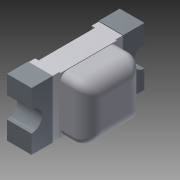
# Autodesk Inventor part: 0603_led
Saved by Autodesk Inventor 2013 (Build 170138000, 138)
## iProperties
Created: 2015-03-28
Part Number: 0603_led
Material: Ogólny
Document SubType Name: Modeling
Designer: terg
Density: 1 g/cm^3
Author: terg
Autodesk Inventor part; units mm, degrees
ref_plane "YZ Plane" through (0, 0, 0) normal (1, 0, 0) x (0, 1, 0)
ref_plane "XZ Plane" through (0, 0, 0) normal (0, 1, 0) x (-1, 0, 0)
ref_plane "XY Plane" through (0, 0, 0) normal (0, 0, 1) x (1, 0, 0)
sketch "Szkic1" plane through (0, 0, 0) normal (1, 0, 0) x (0, 1, 0)
  line L0 (0, 0) -> (1.6, 0)
  line L1 (1.6, 0) -> (1.6, 0.8)
  line L2 (1.6, 0.8) -> (0, 0.8)
  line L3 (0, 0.8) -> (0, 0)
  dimension "d0" = 1.6
  dimension "d1" = 0.8
  constraints: 8 end point, 2 parallel, 1 horizontal, 1 perpendicular
  measures "d0" distance of L2.end L1.end
  measures "d1" distance of L1.end L0.end
extrude "Wyciągnięcie proste1" add sketch "Szkic1" along normal blind 0.3
sketch "Szkic2" plane through (0.3, 0, 0) normal (1, 0, 0) x (0, 0, -1)
  line L0 (0, 0) -> (0, 1.6) projected
  line L1 (0, 1.6) -> (-0.8, 1.6) projected
  line L2 (-0.8, 1.6) -> (-0.8, 0) projected
  line L3 (-0.8, 0) -> (0, 0) projected
  line L4 (-0.8, 1.2) -> (0, 1.2)
  line L5 (0, 1.2) -> (0, 0.4)
  line L6 (0, 0.4) -> (-0.8, 0.4)
  line L7 (-0.8, 0.4) -> (-0.8, 1.2)
  dimension "d4" = 0.4
  dimension "d5" = 0.4
  dimension "d6" = 0
  dimension "d7" = 0
  constraints: 8 end point, 2 parallel, 1 horizontal, 1 perpendicular
  measures "d4" distance between parallel lines of L1 L4
  measures "d5" distance between parallel lines of L3 L6
  measures "d6" distance between parallel lines of L0 L5
  measures "d7" distance between parallel lines of L2 L7
extrude "Wyciągnięcie proste2" add sketch "Szkic2" along normal blind 0.4 contours L6 L2 L4 L0
sketch "Szkic4" plane through (0, 0, 0) normal (-1, 0, 0) x (0, 0, 1)
  line L0 (0.8, 1.6) -> (0.8, 0) projected
  line L1 (0, 1.6) -> (0.8, 1.6)
  line L2 (0.8, 1.6) -> (0.8, 1.2)
  line L3 (0.8, 1.2) -> (0, 1.2)
  line L4 (0, 1.2) -> (0, 1.6)
  line L5 (0, 0) -> (0.8, 0)
  line L6 (0.8, 0) -> (0.8, 0.4)
  line L7 (0.8, 0.4) -> (0, 0.4)
  line L8 (0, 0.4) -> (0, 0)
  dimension "d10" = 0.4
  dimension "d11" = 0.4
  constraints: 16 end point, 4 parallel, 2 horizontal, 2 perpendicular, 2 point on line
  measures "d10" distance of L1.end L2.end
  measures "d11" distance of L6.end L5.end
extrude "Wyciągnięcie proste3" add sketch "Szkic4" along normal blind 0.05
sketch "Szkic8" plane through (0.7, 0, 0) normal (1, 0, 0) x (0, 0, -1)
  line L0 (0, 1.2) -> (-0.8, 1.2) projected
  line L1 (-0.8, 0.4) -> (0, 0.4) projected
  line L2 (0, 0.4) -> (0, 1.2) projected
  line L3 (-0.01, 1.2) -> (0, 1.2)
  line L4 (0, 1.2) -> (0, 0.4)
  line L5 (0, 0.4) -> (-0.01, 0.4)
  line L6 (-0.01, 0.4) -> (-0.01, 1.2)
  line L7 (-0.8, 1.2) -> (-0.79, 1.2)
  line L8 (-0.79, 1.2) -> (-0.79, 0.4)
  line L9 (-0.79, 0.4) -> (-0.8, 0.4)
  line L10 (-0.8, 0.4) -> (-0.8, 1.2)
  point P0 (0, 0)
  dimension "d20" = 0.01
  dimension "d21" = 0
  dimension "d22" = 0.01
  constraints: 16 end point, 4 parallel, 3 point on line, 2 horizontal, 2 perpendicular
  measures "d20" distance of L4.end L5.end
  measures "d21" distance between parallel lines of L2 L4
  measures "d22" distance of L8.end L9.end
extrude "Wyciągnięcie proste7" cut sketch "Szkic8" against normal blind 0.39 contours L2 L1 L6 L0 | L8 L1 L10 L0
sketch "Szkic9" plane through (0.3, 0, 0) normal (1, 0, 0) x (0, 0, -1)
  line L0 (-0.8, 0) -> (0, 0) projected
  line L1 (-0.8, 1.2) -> (0, 1.2) projected
  line L2 (0, 1.2) -> (0, 1.6) projected
  line L3 (0, 1.6) -> (-0.8, 1.6) projected
  line L4 (-0.8, 1.6) -> (-0.8, 1.2) projected
  point P0 (-0.4, 0)
  point P1 (-0.4, 1.6)
  constraints: 2 midpoint
hole "Otwór1" at (0.3, 0, 0.4) at (0.3, 1.6, 0.4) direction (-1, 0, 0) diameter 0.3 depth 8
sketch "Szkic10" plane through (0.3, 0, 0) normal (1, 0, 0) x (0, 0, -1)
  line L0 (-0.8, 1.6) -> (-0.8, 1.2) projected
  line L1 (-0.8, 1.2) -> (0, 1.2) projected
  line L2 (0, 1.2) -> (0, 1.6) projected
  arc A0 (-0.25, 0) -> (-0.55, 0) centre (-0.4, 0) ccw projected
  line L3 (-0.25, 0) -> (0, 0) projected
  line L4 (0, 0) -> (0, 0.4) projected
  line L5 (0, 0.4) -> (-0.8, 0.4) projected
  line L6 (-0.8, 0.4) -> (-0.8, 0) projected
  line L7 (-0.8, 0) -> (-0.55, 0) projected
  line L8 (-0.8, 1.3) -> (0, 1.3)
  line L9 (0, 1.3) -> (0, 1.2)
  line L10 (0, 1.2) -> (-0.8, 1.2)
  line L11 (-0.8, 1.2) -> (-0.8, 1.3)
  line L12 (-0.8, 0.4) -> (0, 0.4)
  line L13 (0, 0.4) -> (0, 0.3)
  line L14 (0, 0.3) -> (-0.8, 0.3)
  line L15 (-0.8, 0.3) -> (-0.8, 0.4)
  dimension "d32" = 0.1
  dimension "d33" = 0.1
  dimension "d34" = 0
  constraints: 16 end point, 4 parallel, 3 point on line, 2 horizontal, 2 perpendicular
  measures "d32" distance of L8.end L9.end
  measures "d33" distance of L12.end L13.end
  measures "d34" distance between parallel lines of L1 L10
extrude "Wyciągnięcie proste8" cut sketch "Szkic10" against normal blind 0.01 contours L8 L2 L1 L0 | L14 L6 L5 L4
fillet "Zaokrąglenie1" radius 0.1 4 edges at (0.505, 1.2, 0.79) (0.505, 0.4, 0.79) (0.505, 1.2, 0.01) (0.505, 0.4, 0.01)
fillet "Zaokrąglenie2" radius 0.2 8 edges at (0.7, 0.4293, 0.7607) (0.7, 0.4, 0.4) (0.7, 0.4293, 0.0393) (0.7, 0.8, 0.01) (0.7, 1.1707, 0.0393) (0.7, 1.2, 0.4) (0.7, 1.1707, 0.7607) (0.7, 0.8, 0.79)
sketch "Szkic11" plane through (0, 0.4, 0.8) normal (0, 0, 1) x (1, 0, 0)
  line L0 (-0.05, 0.8) -> (-0.05, 1.2) projected
  line L1 (0.3, -0.1) -> (-0.05, -0.1)
  line L2 (-0.05, -0.1) -> (-0.05, -0.4)
  line L3 (-0.05, -0.4) -> (0.3, -0.4)
  line L4 (0.3, -0.4) -> (0.3, -0.1)
  line L5 (0.3, 1.2) -> (-0.05, 1.2)
  line L6 (-0.05, 1.2) -> (-0.05, 0.9)
  line L7 (-0.05, 0.9) -> (0.3, 0.9)
  line L8 (0.3, 0.9) -> (0.3, 1.2)
  point P0 (0.29, 0.9)
  point P1 (0, -0.4)
  dimension "d39" = 0
  constraints: 16 end point, 4 parallel, 2 horizontal, 2 perpendicular, 1 point on line
  measures "d39" distance from line of point (0.29, 0.9) L7
extrude "Wyciągnięcie proste9" add sketch "Szkic11" along normal blind 0.01
sketch "Szkic12" plane through (0, 0.4, 0) normal (0, 0, -1) x (-1, 0, 0)
  line L0 (0.05, 1.2) -> (0.05, 0.8) projected
  line L1 (-0.3, 1.2) -> (0.05, 1.2)
  line L2 (0.05, 1.2) -> (0.05, 0.9)
  line L3 (0.05, 0.9) -> (-0.3, 0.9)
  line L4 (-0.3, 0.9) -> (-0.3, 1.2)
  line L5 (-0.3, -0.1) -> (0.05, -0.1)
  line L6 (0.05, -0.1) -> (0.05, -0.4)
  line L7 (0.05, -0.4) -> (-0.3, -0.4)
  line L8 (-0.3, -0.4) -> (-0.3, -0.1)
  point P0 (-0.3, 0.9)
  point P1 (0, -0.4)
  dimension "d42" = 0
  constraints: 16 end point, 4 parallel, 2 horizontal, 2 perpendicular, 1 point on line
  measures "d42" distance from line of point (-0.3, 0.9) L3
extrude "Wyciągnięcie proste10" add sketch "Szkic12" along normal blind 0.01
